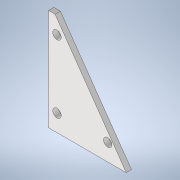
# Autodesk Inventor part: shooter guid
Saved by Autodesk Inventor 2021 (Build 250183000, 183)
## iProperties
Created: 2021-03-18
Part Number: shooter guid
Material: Generic
Document SubType Name: Modeling
Designer: deli
Density: 1 g/cm^3
Appearance: Default
Author: deli
Autodesk Inventor part; units mm, degrees
ref_plane "YZ Plane" through (0, 0, 0) normal (1, 0, 0) x (0, 1, 0)
ref_plane "XZ Plane" through (0, 0, 0) normal (0, 1, 0) x (-1, 0, 0)
ref_plane "XY Plane" through (0, 0, 0) normal (0, 0, 1) x (1, 0, 0)
sketch "Sketch1" plane through (0, 0, 0) normal (0, 0, 1) x (1, 0, 0)
  line L0 (0, 0) -> (-96, 0) projected
  line L1 (-96, 0) -> (-96, -48) projected
  line L2 (0, -48) -> (-96, -48) projected
  line L3 (0, 0) -> (0, -48) projected
  line L4 (-31.0711, -33.8995) -> (-30.5858, -33.4142) projected
  arc A0 (-33.8995, -31.0711) -> (-31.0711, -33.8995) centre (-32.4853, -32.4853) ccw projected
  line L5 (-33.8995, -31.0711) -> (-33.4142, -30.5858) projected
  arc A1 (-30.5858, -33.4142) -> (-33.4142, -30.5858) centre (-32, -32) ccw projected
  circle A2 centre (-16, -40) radius 2 projected
  circle A3 centre (-32, -40) radius 2 projected
  arc A4 (-38.5858, -30.5858) -> (-41.4142, -33.4142) centre (-40, -32) ccw projected
  line L6 (-38.1005, -31.0711) -> (-38.5858, -30.5858) projected
  arc A5 (-40.9289, -33.8995) -> (-38.1005, -31.0711) centre (-39.5147, -32.4853) ccw projected
  line L7 (-40.9289, -33.8995) -> (-41.4142, -33.4142) projected
  arc A6 (-41.4142, -14.5858) -> (-38.5858, -17.4142) centre (-40, -16) ccw projected
  line L8 (-40.9289, -14.1005) -> (-41.4142, -14.5858) projected
  arc A7 (-38.1005, -16.9289) -> (-40.9289, -14.1005) centre (-39.5147, -15.5147) ccw projected
  line L9 (-38.1005, -16.9289) -> (-38.5858, -17.4142) projected
  circle A8 centre (-40, -8) radius 2 projected
  arc A9 (-9.4142, -17.4142) -> (-6.5858, -14.5858) centre (-8, -16) ccw projected
  line L10 (-9.8995, -16.9289) -> (-9.4142, -17.4142) projected
  arc A10 (-7.0711, -14.1005) -> (-9.8995, -16.9289) centre (-8.4853, -15.5147) ccw projected
  line L11 (-7.0711, -14.1005) -> (-6.5858, -14.5858) projected
  circle A11 centre (-24, -24) radius 7 projected
  line L12 (-22, -8) -> (-22, -12.6863) projected
  arc A12 (-26, -12.6863) -> (-22, -12.6863) centre (-24, -12.6863) ccw projected
  line L13 (-26, -8) -> (-26, -12.6863) projected
  arc A13 (-22, -8) -> (-26, -8) centre (-24, -8) ccw projected
  line L14 (-11.3137, -26) -> (-12.6863, -26) projected
  arc A14 (-12.6863, -22) -> (-12.6863, -26) centre (-12.6863, -24) ccw projected
  line L15 (-12.6863, -22) -> (-11.3137, -22) projected
  arc A15 (-11.3137, -26) -> (-11.3137, -22) centre (-11.3137, -24) ccw projected
  line L16 (-26, -40) -> (-26, -35.3137) projected
  arc A16 (-22, -35.3137) -> (-26, -35.3137) centre (-24, -35.3137) ccw projected
  line L17 (-22, -40) -> (-22, -35.3137) projected
  arc A17 (-26, -40) -> (-22, -40) centre (-24, -40) ccw projected
  line L18 (-36.6863, -22) -> (-35.3137, -22) projected
  arc A18 (-35.3137, -26) -> (-35.3137, -22) centre (-35.3137, -24) ccw projected
  line L19 (-35.3137, -26) -> (-36.6863, -26) projected
  arc A19 (-36.6863, -22) -> (-36.6863, -26) centre (-36.6863, -24) ccw projected
  circle A20 centre (-16, -8) radius 2 projected
  circle A21 centre (-8, -8) radius 2 projected
  arc A22 (-6.5858, -33.4142) -> (-9.4142, -30.5858) centre (-8, -32) ccw projected
  line L20 (-7.0711, -33.8995) -> (-6.5858, -33.4142) projected
  arc A23 (-9.8995, -31.0711) -> (-7.0711, -33.8995) centre (-8.4853, -32.4853) ccw projected
  line L21 (-9.8995, -31.0711) -> (-9.4142, -30.5858) projected
  circle A24 centre (-8, -40) radius 2 projected
  circle A25 centre (-32, -8) radius 2 projected
  circle A26 centre (-40, -40) radius 2 projected
  line L22 (-14.1005, -31.0711) -> (-14.5858, -30.5858) projected
  arc A27 (-16.9289, -33.8995) -> (-14.1005, -31.0711) centre (-15.5147, -32.4853) ccw projected
  line L23 (-16.9289, -33.8995) -> (-17.4142, -33.4142) projected
  arc A28 (-14.5858, -30.5858) -> (-17.4142, -33.4142) centre (-16, -32) ccw projected
  arc A29 (-17.4142, -14.5858) -> (-14.5858, -17.4142) centre (-16, -16) ccw projected
  line L24 (-16.9289, -14.1005) -> (-17.4142, -14.5858) projected
  arc A30 (-14.1005, -16.9289) -> (-16.9289, -14.1005) centre (-15.5147, -15.5147) ccw projected
  line L25 (-14.1005, -16.9289) -> (-14.5858, -17.4142) projected
  line L26 (-31.0711, -14.1005) -> (-30.5858, -14.5858) projected
  arc A31 (-33.4142, -17.4142) -> (-30.5858, -14.5858) centre (-32, -16) ccw projected
  line L27 (-33.8995, -16.9289) -> (-33.4142, -17.4142) projected
  arc A32 (-31.0711, -14.1005) -> (-33.8995, -16.9289) centre (-32.4853, -15.5147) ccw projected
  line L28 (-79.0711, -14.1005) -> (-78.5858, -14.5858) projected
  arc A33 (-81.4142, -17.4142) -> (-78.5858, -14.5858) centre (-80, -16) ccw projected
  line L29 (-81.8995, -16.9289) -> (-81.4142, -17.4142) projected
  arc A34 (-79.0711, -14.1005) -> (-81.8995, -16.9289) centre (-80.4853, -15.5147) ccw projected
  circle A35 centre (-88, -40) radius 2 projected
  circle A36 centre (-80, -8) radius 2 projected
  line L30 (-84.6863, -22) -> (-83.3137, -22) projected
  arc A37 (-83.3137, -26) -> (-83.3137, -22) centre (-83.3137, -24) ccw projected
  line L31 (-83.3137, -26) -> (-84.6863, -26) projected
  arc A38 (-84.6863, -22) -> (-84.6863, -26) centre (-84.6863, -24) ccw projected
  line L32 (-74, -40) -> (-74, -35.3137) projected
  arc A39 (-70, -35.3137) -> (-74, -35.3137) centre (-72, -35.3137) ccw projected
  line L33 (-70, -40) -> (-70, -35.3137) projected
  arc A40 (-74, -40) -> (-70, -40) centre (-72, -40) ccw projected
  line L34 (-70, -8) -> (-70, -12.6863) projected
  arc A41 (-74, -12.6863) -> (-70, -12.6863) centre (-72, -12.6863) ccw projected
  line L35 (-74, -8) -> (-74, -12.6863) projected
  arc A42 (-70, -8) -> (-74, -8) centre (-72, -8) ccw projected
  circle A43 centre (-72, -24) radius 7 projected
  circle A44 centre (-88, -8) radius 2 projected
  arc A45 (-89.4142, -14.5858) -> (-86.5858, -17.4142) centre (-88, -16) ccw projected
  line L36 (-88.9289, -14.1005) -> (-89.4142, -14.5858) projected
  arc A46 (-86.1005, -16.9289) -> (-88.9289, -14.1005) centre (-87.5147, -15.5147) ccw projected
  line L37 (-86.1005, -16.9289) -> (-86.5858, -17.4142) projected
  arc A47 (-86.5858, -30.5858) -> (-89.4142, -33.4142) centre (-88, -32) ccw projected
  line L38 (-86.1005, -31.0711) -> (-86.5858, -30.5858) projected
  arc A48 (-88.9289, -33.8995) -> (-86.1005, -31.0711) centre (-87.5147, -32.4853) ccw projected
  line L39 (-88.9289, -33.8995) -> (-89.4142, -33.4142) projected
  circle A49 centre (-80, -40) radius 2 projected
  line L40 (-79.0711, -33.8995) -> (-78.5858, -33.4142) projected
  arc A50 (-81.8995, -31.0711) -> (-79.0711, -33.8995) centre (-80.4853, -32.4853) ccw projected
  line L41 (-81.8995, -31.0711) -> (-81.4142, -30.5858) projected
  arc A51 (-78.5858, -33.4142) -> (-81.4142, -30.5858) centre (-80, -32) ccw projected
  line L42 (-55.0711, -14.1005) -> (-54.5858, -14.5858) projected
  arc A52 (-57.4142, -17.4142) -> (-54.5858, -14.5858) centre (-56, -16) ccw projected
  line L43 (-57.8995, -16.9289) -> (-57.4142, -17.4142) projected
  arc A53 (-55.0711, -14.1005) -> (-57.8995, -16.9289) centre (-56.4853, -15.5147) ccw projected
  circle A54 centre (-64, -40) radius 2 projected
  circle A55 centre (-56, -8) radius 2 projected
  line L44 (-60.6863, -22) -> (-59.3137, -22) projected
  arc A56 (-59.3137, -26) -> (-59.3137, -22) centre (-59.3137, -24) ccw projected
  line L45 (-59.3137, -26) -> (-60.6863, -26) projected
  arc A57 (-60.6863, -22) -> (-60.6863, -26) centre (-60.6863, -24) ccw projected
  line L46 (-50, -40) -> (-50, -35.3137) projected
  arc A58 (-46, -35.3137) -> (-50, -35.3137) centre (-48, -35.3137) ccw projected
  line L47 (-46, -40) -> (-46, -35.3137) projected
  arc A59 (-50, -40) -> (-46, -40) centre (-48, -40) ccw projected
  line L48 (-46, -8) -> (-46, -12.6863) projected
  arc A60 (-50, -12.6863) -> (-46, -12.6863) centre (-48, -12.6863) ccw projected
  line L49 (-50, -8) -> (-50, -12.6863) projected
  arc A61 (-46, -8) -> (-50, -8) centre (-48, -8) ccw projected
  circle A62 centre (-48, -24) radius 7 projected
  circle A63 centre (-64, -8) radius 2 projected
  arc A64 (-65.4142, -14.5858) -> (-62.5858, -17.4142) centre (-64, -16) ccw projected
  line L50 (-64.9289, -14.1005) -> (-65.4142, -14.5858) projected
  arc A65 (-62.1005, -16.9289) -> (-64.9289, -14.1005) centre (-63.5147, -15.5147) ccw projected
  line L51 (-62.1005, -16.9289) -> (-62.5858, -17.4142) projected
  arc A66 (-62.5858, -30.5858) -> (-65.4142, -33.4142) centre (-64, -32) ccw projected
  line L52 (-62.1005, -31.0711) -> (-62.5858, -30.5858) projected
  arc A67 (-64.9289, -33.8995) -> (-62.1005, -31.0711) centre (-63.5147, -32.4853) ccw projected
  line L53 (-64.9289, -33.8995) -> (-65.4142, -33.4142) projected
  circle A68 centre (-56, -40) radius 2 projected
  line L54 (-55.0711, -33.8995) -> (-54.5858, -33.4142) projected
  arc A69 (-57.8995, -31.0711) -> (-55.0711, -33.8995) centre (-56.4853, -32.4853) ccw projected
  line L55 (-57.8995, -31.0711) -> (-57.4142, -30.5858) projected
  arc A70 (-54.5858, -33.4142) -> (-57.4142, -30.5858) centre (-56, -32) ccw projected
  line L56 (6.0209, -101.2733) -> (-90.3399, 36.3443) projected
  line L57 (-68, 0) -> (-68, -48)
  circle A71 centre (-64, -8) radius 2.15
  circle A72 centre (-64, -40) radius 2.15
  circle A73 centre (-48, -40) radius 2
  circle A74 centre (-48, -40) radius 2.15
  point P0 (-64.8914, 0)
  point P1 (-31.2814, -48)
  dimension "d0" = 4
  dimension "d3" = 0.15
  dimension "d4" = 0.15
  dimension "d5" = 0.15
  constraints: 4 centre point, 2 end point, 1 coincident, 1 concentric, 1 point on line, 1 vertical
  measures "d0" distance from line of A63.centre L57
  measures "d3" radial gap between concentric circles of A63 A71
  measures "d4" radial gap between concentric circles of A54 A72
  measures "d5" radial gap between concentric circles of A73 A74
extrude "Extrusion1" add sketch "Sketch1" along normal blind 2.5 contours L0 L56 L42 A53 L43 A52 A62 L2 L57 A43 | A43 L57 | L56 A52 L43 A53 L42 | L56 A62 | A26 | L44 A56 L45 A57 | L46 A58 L47 A74 | L50 A65 L51 A64 | L52 A67 L53 A66 | A68 | A69 L55 A70 L54 picked at (-67.5821, -25.5419) picked at (-50.3108, -23.4962)
sketch "Sketch2" plane through (-64.8914, 0, 2.5) normal (0.8192, 0.5736, 0) x (0, 0, -1)
  line L0 (2.5, -58.5972) -> (2.5, 0) projected
  line L1 (2.5, 0) -> (0, 0) projected
  line L2 (0, -58.5972) -> (0, 0) projected
  line L3 (2.5, -58.5972) -> (0, -58.5972) projected
  line L4 (-26.6333, 19.2846) -> (36.9911, 19.2846)
  line L5 (36.9911, 19.2846) -> (36.9911, -71.9639)
  line L6 (36.9911, -71.9639) -> (-26.6333, -71.9639)
  line L7 (-26.6333, -71.9639) -> (-26.6333, 19.2846)
  point P0 (2.5, -37.2202)
  constraints: 8 end point, 2 parallel, 1 horizontal, 1 perpendicular
body "Solid1"
